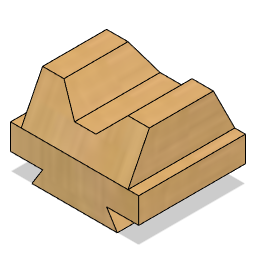
Assignment 1 (Autodesk Fusion 360 design; units mm, degrees)
Autodesk Fusion 360 part; units mm, degrees
sketch "Sketch1" plane through (0, 0, 0) normal (0, 0, 1) x (1, 0, 0)
  line L0 (0, 0) -> (40, 0)
  line L1 (0, 0) -> (5, 8)
  line L2 (35, 8) -> (40, 0)
  line L3 (5, 8) -> (-10, 8)
  line L4 (-10, 8) -> (-10, 20)
  line L5 (-10, 20) -> (50, 20)
  line L6 (50, 20) -> (50, 8)
  line L7 (50, 8) -> (35, 8)
  line L8 (-5, 20) -> (-5, 40)
  line L9 (-5, 40) -> (5, 40)
  line L10 (15, 30) -> (25, 30)
  line L11 (35, 40) -> (45, 40)
  line L12 (45, 40) -> (45, 20)
  line L13 (5, 40) -> (15, 30)
  line L14 (35, 40) -> (25, 30)
  dimension "d1" = 40
  dimension "d2" = 30
  dimension "d5" = 12
  dimension "d8" = 60
  dimension "d9" = 5
  dimension "d10" = 5
  dimension "d11" = 10
  dimension "d14" = 10
  dimension "d15" = 10
  dimension "d16" = 20
  dimension "d17" = 8
  constraint coincident L0.start L1.start
  constraint horizontal L0
  constraint perpendicular L4 L5
  constraint perpendicular L5 L6
  constraint perpendicular L6 L7
  constraint equal L3 L7
  constraint equal L1 L2
  constraint equal L4 L6
  constraint perpendicular L3 L4
  constraint coincident L5 L8.start
  constraint perpendicular L5 L8
  constraint perpendicular L8 L9
  constraint coincident L5 L12.end
  constraint perpendicular L5 L12
  constraint equal L8 L12
  constraint equal L9 L11
  constraint equal L13 L14
  constraint perpendicular L11 L12
  measures "d1" distance of L0.start L0.end
  measures "d2" distance of L1.end L2.start
  measures "d5" distance of L3.end L4.end
  measures "d8" distance of L4.end L5.end
  measures "d9" distance of L4 L8
  measures "d10" distance of L6 L12
  measures "d11" distance of L8.end L9.end
  measures "d14" distance of L10.start L10.end
  measures "d15" distance of L5 L10
  measures "d16" distance of L8.start L8.end
  measures "d17" distance of L0 L3
extrude "Extrude1" add sketch "Sketch1" against normal blind 50
chamfer "Chamfer1" distance 10 distance2 20 1 edges at (0, 40, 0) measured on face at (-1.6667, 40, -16.6667)
chamfer "Chamfer2" distance 20 distance2 10 1 edges at (40, 40, -50) measured on face at (18.3333, 15.3333, -50)
